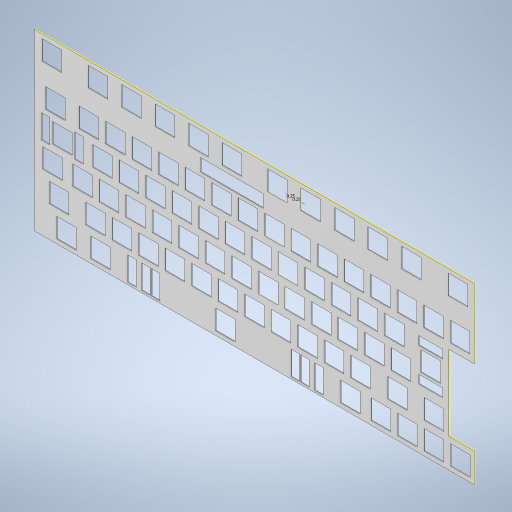
# Autodesk Inventor part: Plate
Saved by Autodesk Inventor 2024 (Build 280153000, 153)
## iProperties
Created: 2024-06-26
Part Number: Plate
Material: PET Plastic
Document SubType Name: Modeling
Designer: adam
Density: 1.541 g/cm^3
Appearance: Smooth - White
Author: adam
Autodesk Inventor part; units mm, degrees
(part 1 of 2)
ref_plane "YZ Plane" through (0, 0, 0) normal (1, 0, 0) x (0, 1, 0)
ref_plane "XZ Plane" through (0, 0, 0) normal (0, 1, 0) x (-1, 0, 0)
ref_plane "XY Plane" through (0, 0, 0) normal (0, 0, 1) x (1, 0, 0)
sketch "Keyswitch cut positions" plane through (0, 0, 0) normal (0, 0, 1) x (1, 0, 0)
  line L0 (0, 0) -> (315, 0)
  line L1 (315, -125) -> (0, -125)
  line L2 (0, -125) -> (0, 0)
  line L3 (5.475, -2.975) -> (19.525, -2.975)
  line L4 (19.525, -2.975) -> (19.525, -17.025)
  line L5 (19.525, -17.025) -> (5.475, -17.025)
  line L6 (5.475, -17.025) -> (5.475, -2.975)
  line L7 (5.475, -2.975) -> (19.525, -17.025) construction
  line L8 (19.525, -2.975) -> (5.475, -17.025) construction
  line L9 (38.475, -2.975) -> (52.525, -2.975)
  line L10 (52.525, -2.975) -> (52.525, -17.025)
  line L11 (52.525, -17.025) -> (38.475, -17.025)
  line L12 (38.475, -17.025) -> (38.475, -2.975)
  line L13 (38.475, -2.975) -> (52.525, -17.025) construction
  line L14 (52.525, -2.975) -> (38.475, -17.025) construction
  line L15 (62.475, -2.975) -> (76.525, -2.975)
  line L16 (76.525, -2.975) -> (76.525, -17.025)
  line L17 (76.525, -17.025) -> (62.475, -17.025)
  line L18 (62.475, -17.025) -> (62.475, -2.975)
  line L19 (62.475, -2.975) -> (76.525, -17.025) construction
  line L20 (76.525, -2.975) -> (62.475, -17.025) construction
  line L21 (86.475, -2.975) -> (100.525, -2.975)
  line L22 (100.525, -2.975) -> (100.525, -17.025)
  line L23 (100.525, -17.025) -> (86.475, -17.025)
  line L24 (86.475, -17.025) -> (86.475, -2.975)
  line L25 (86.475, -2.975) -> (100.525, -17.025) construction
  line L26 (100.525, -2.975) -> (86.475, -17.025) construction
  line L27 (110.475, -2.975) -> (124.525, -2.975)
  line L28 (124.525, -2.975) -> (124.525, -17.025)
  line L29 (124.525, -17.025) -> (110.475, -17.025)
  line L30 (110.475, -17.025) -> (110.475, -2.975)
  line L31 (110.475, -2.975) -> (124.525, -17.025) construction
  line L32 (124.525, -2.975) -> (110.475, -17.025) construction
  line L33 (134.475, -2.975) -> (148.525, -2.975)
  line L34 (148.525, -2.975) -> (148.525, -17.025)
  line L35 (148.525, -17.025) -> (134.475, -17.025)
  line L36 (134.475, -17.025) -> (134.475, -2.975)
  line L37 (134.475, -2.975) -> (148.525, -17.025) construction
  line L38 (148.525, -2.975) -> (134.475, -17.025) construction
  line L39 (166.975, -2.975) -> (181.025, -2.975)
  line L40 (181.025, -2.975) -> (181.025, -17.025)
  line L41 (181.025, -17.025) -> (166.975, -17.025)
  line L42 (166.975, -17.025) -> (166.975, -2.975)
  line L43 (166.975, -2.975) -> (181.025, -17.025) construction
  line L44 (181.025, -2.975) -> (166.975, -17.025) construction
  line L45 (190.975, -2.975) -> (205.025, -2.975)
  line L46 (205.025, -2.975) -> (205.025, -17.025)
  line L47 (205.025, -17.025) -> (190.975, -17.025)
  line L48 (190.975, -17.025) -> (190.975, -2.975)
  line L49 (190.975, -2.975) -> (205.025, -17.025) construction
  line L50 (205.025, -2.975) -> (190.975, -17.025) construction
  line L51 (214.975, -2.975) -> (229.025, -2.975)
  line L52 (229.025, -2.975) -> (229.025, -17.025)
  line L53 (229.025, -17.025) -> (214.975, -17.025)
  line L54 (214.975, -17.025) -> (214.975, -2.975)
  line L55 (214.975, -2.975) -> (229.025, -17.025) construction
  line L56 (229.025, -2.975) -> (214.975, -17.025) construction
  line L57 (238.975, -2.975) -> (253.025, -2.975)
  line L58 (253.025, -2.975) -> (253.025, -17.025)
  line L59 (253.025, -17.025) -> (238.975, -17.025)
  line L60 (238.975, -17.025) -> (238.975, -2.975)
  line L61 (238.975, -2.975) -> (253.025, -17.025) construction
  line L62 (253.025, -2.975) -> (238.975, -17.025) construction
  line L63 (262.975, -2.975) -> (277.025, -2.975)
  line L64 (277.025, -2.975) -> (277.025, -17.025)
  line L65 (277.025, -17.025) -> (262.975, -17.025)
  line L66 (262.975, -17.025) -> (262.975, -2.975)
  line L67 (262.975, -2.975) -> (277.025, -17.025) construction
  line L68 (277.025, -2.975) -> (262.975, -17.025) construction
  line L69 (296.475, -2.975) -> (310.525, -2.975)
  line L70 (310.525, -2.975) -> (310.525, -17.025)
  line L71 (310.525, -17.025) -> (296.475, -17.025)
  line L72 (296.475, -17.025) -> (296.475, -2.975)
  line L73 (296.475, -2.975) -> (310.525, -17.025) construction
  line L74 (310.525, -2.975) -> (296.475, -17.025) construction
  line L75 (7.975, -31.475) -> (22.025, -31.475)
  line L76 (22.025, -31.475) -> (22.025, -45.525)
  line L77 (22.025, -45.525) -> (7.975, -45.525)
  line L78 (7.975, -45.525) -> (7.975, -31.475)
  line L79 (7.975, -31.475) -> (22.025, -45.525) construction
  line L80 (22.025, -31.475) -> (7.975, -45.525) construction
  line L81 (31.975, -31.475) -> (46.025, -31.475)
  line L82 (46.025, -31.475) -> (46.025, -45.525)
  line L83 (46.025, -45.525) -> (31.975, -45.525)
  line L84 (31.975, -45.525) -> (31.975, -31.475)
  line L85 (31.975, -31.475) -> (46.025, -45.525) construction
  line L86 (46.025, -31.475) -> (31.975, -45.525) construction
  line L87 (50.975, -31.475) -> (65.025, -31.475)
  line L88 (65.025, -31.475) -> (65.025, -45.525)
  line L89 (65.025, -45.525) -> (50.975, -45.525)
  line L90 (50.975, -45.525) -> (50.975, -31.475)
  line L91 (50.975, -31.475) -> (65.025, -45.525) construction
  line L92 (65.025, -31.475) -> (50.975, -45.525) construction
  line L93 (69.975, -31.475) -> (84.025, -31.475)
  line L94 (84.025, -31.475) -> (84.025, -45.525)
  line L95 (84.025, -45.525) -> (69.975, -45.525)
  line L96 (69.975, -45.525) -> (69.975, -31.475)
  line L97 (69.975, -31.475) -> (84.025, -45.525) construction
  line L98 (84.025, -31.475) -> (69.975, -45.525) construction
  line L99 (88.975, -31.475) -> (103.025, -31.475)
  line L100 (103.025, -31.475) -> (103.025, -45.525)
  line L101 (103.025, -45.525) -> (88.975, -45.525)
  line L102 (88.975, -45.525) -> (88.975, -31.475)
  line L103 (88.975, -31.475) -> (103.025, -45.525) construction
  line L104 (103.025, -31.475) -> (88.975, -45.525) construction
  line L105 (107.975, -31.475) -> (122.025, -31.475)
  line L106 (122.025, -31.475) -> (122.025, -45.525)
  line L107 (122.025, -45.525) -> (107.975, -45.525)
  line L108 (107.975, -45.525) -> (107.975, -31.475)
  line L109 (107.975, -31.475) -> (122.025, -45.525) construction
  line L110 (122.025, -31.475) -> (107.975, -45.525) construction
  line L111 (126.975, -31.475) -> (141.025, -31.475)
  line L112 (141.025, -31.475) -> (141.025, -45.525)
  line L113 (141.025, -45.525) -> (126.975, -45.525)
  line L114 (126.975, -45.525) -> (126.975, -31.475)
  line L115 (126.975, -31.475) -> (141.025, -45.525) construction
  line L116 (141.025, -31.475) -> (126.975, -45.525) construction
  line L117 (145.975, -31.475) -> (160.025, -31.475)
  line L118 (160.025, -31.475) -> (160.025, -45.525)
  line L119 (160.025, -45.525) -> (145.975, -45.525)
  line L120 (145.975, -45.525) -> (145.975, -31.475)
  line L121 (145.975, -31.475) -> (160.025, -45.525) construction
  line L122 (160.025, -31.475) -> (145.975, -45.525) construction
  line L123 (164.975, -31.475) -> (179.025, -31.475)
  line L124 (179.025, -31.475) -> (179.025, -45.525)
  line L125 (179.025, -45.525) -> (164.975, -45.525)
  line L126 (164.975, -45.525) -> (164.975, -31.475)
  line L127 (164.975, -31.475) -> (179.025, -45.525) construction
  line L128 (179.025, -31.475) -> (164.975, -45.525) construction
  line L129 (183.975, -31.475) -> (198.025, -31.475)
  line L130 (198.025, -31.475) -> (198.025, -45.525)
  line L131 (198.025, -45.525) -> (183.975, -45.525)
  line L132 (183.975, -45.525) -> (183.975, -31.475)
  line L133 (183.975, -31.475) -> (198.025, -45.525) construction
  line L134 (198.025, -31.475) -> (183.975, -45.525) construction
  line L135 (202.975, -31.475) -> (217.025, -31.475)
  line L136 (217.025, -31.475) -> (217.025, -45.525)
  line L137 (217.025, -45.525) -> (202.975, -45.525)
  line L138 (202.975, -45.525) -> (202.975, -31.475)
  line L139 (202.975, -31.475) -> (217.025, -45.525) construction
  line L140 (217.025, -31.475) -> (202.975, -45.525) construction
  line L141 (221.975, -31.475) -> (236.025, -31.475)
  line L142 (236.025, -31.475) -> (236.025, -45.525)
  line L143 (236.025, -45.525) -> (221.975, -45.525)
  line L144 (221.975, -45.525) -> (221.975, -31.475)
  line L145 (221.975, -31.475) -> (236.025, -45.525) construction
  line L146 (236.025, -31.475) -> (221.975, -45.525) construction
  line L147 (240.975, -31.475) -> (255.025, -31.475)
  line L148 (255.025, -31.475) -> (255.025, -45.525)
  line L149 (255.025, -45.525) -> (240.975, -45.525)
  line L150 (240.975, -45.525) -> (240.975, -31.475)
  line L151 (240.975, -31.475) -> (255.025, -45.525) construction
  line L152 (255.025, -31.475) -> (240.975, -45.525) construction
  line L153 (259.975, -31.475) -> (274.025, -31.475)
  line L154 (274.025, -31.475) -> (274.025, -45.525)
  line L155 (274.025, -45.525) -> (259.975, -45.525)
  line L156 (259.975, -45.525) -> (259.975, -31.475)
  line L157 (259.975, -31.475) -> (274.025, -45.525) construction
  line L158 (274.025, -31.475) -> (259.975, -45.525) construction
  line L159 (278.975, -31.475) -> (293.025, -31.475)
  line L160 (293.025, -31.475) -> (293.025, -45.525)
  line L161 (293.025, -45.525) -> (278.975, -45.525)
  line L162 (278.975, -45.525) -> (278.975, -31.475)
  line L163 (278.975, -31.475) -> (293.025, -45.525) construction
  line L164 (293.025, -31.475) -> (278.975, -45.525) construction
  line L165 (297.975, -31.475) -> (312.025, -31.475)
  line L166 (312.025, -31.475) -> (312.025, -45.525)
  line L167 (312.025, -45.525) -> (297.975, -45.525)
  line L168 (297.975, -45.525) -> (297.975, -31.475)
  line L169 (297.975, -31.475) -> (312.025, -45.525) construction
  line L170 (312.025, -31.475) -> (297.975, -45.525) construction
  line L171 (12.975, -50.575) -> (27.025, -50.575)
  line L172 (27.025, -50.575) -> (27.025, -64.625)
  line L173 (27.025, -64.625) -> (12.975, -64.625)
  line L174 (12.975, -64.625) -> (12.975, -50.575)
  line L175 (12.975, -50.575) -> (27.025, -64.625) construction
  line L176 (27.025, -50.575) -> (12.975, -64.625) construction
  line L177 (41.725, -50.575) -> (55.775, -50.575)
  line L178 (55.775, -50.575) -> (55.775, -64.625)
  line L179 (55.775, -64.625) -> (41.725, -64.625)
  line L180 (41.725, -64.625) -> (41.725, -50.575)
  line L181 (41.725, -50.575) -> (55.775, -64.625) construction
  line L182 (55.775, -50.575) -> (41.725, -64.625) construction
  line L183 (60.725, -50.575) -> (74.775, -50.575)
  line L184 (74.775, -50.575) -> (74.775, -64.625)
  line L185 (74.775, -64.625) -> (60.725, -64.625)
  line L186 (60.725, -64.625) -> (60.725, -50.575)
  line L187 (60.725, -50.575) -> (74.775, -64.625) construction
  line L188 (74.775, -50.575) -> (60.725, -64.625) construction
  line L189 (79.725, -50.575) -> (93.775, -50.575)
  line L190 (93.775, -50.575) -> (93.775, -64.625)
  line L191 (93.775, -64.625) -> (79.725, -64.625)
  line L192 (79.725, -64.625) -> (79.725, -50.575)
  line L193 (79.725, -50.575) -> (93.775, -64.625) construction
  line L194 (93.775, -50.575) -> (79.725, -64.625) construction
  line L195 (98.725, -50.575) -> (112.775, -50.575)
  line L196 (112.775, -50.575) -> (112.775, -64.625)
  line L197 (112.775, -64.625) -> (98.725, -64.625)
  line L198 (98.725, -64.625) -> (98.725, -50.575)
  line L199 (98.725, -50.575) -> (112.775, -64.625) construction
  line L200 (112.775, -50.575) -> (98.725, -64.625) construction
  line L201 (117.725, -50.575) -> (131.775, -50.575)
  line L202 (131.775, -50.575) -> (131.775, -64.625)
  line L203 (131.775, -64.625) -> (117.725, -64.625)
  line L204 (117.725, -64.625) -> (117.725, -50.575)
  line L205 (117.725, -50.575) -> (131.775, -64.625) construction
  line L206 (131.775, -50.575) -> (117.725, -64.625) construction
  line L207 (136.725, -50.575) -> (150.775, -50.575)
  line L208 (150.775, -50.575) -> (150.775, -64.625)
  line L209 (150.775, -64.625) -> (136.725, -64.625)
  line L210 (136.725, -64.625) -> (136.725, -50.575)
  line L211 (136.725, -50.575) -> (150.775, -64.625) construction
  line L212 (150.775, -50.575) -> (136.725, -64.625) construction
  line L213 (155.725, -50.575) -> (169.775, -50.575)
  line L214 (169.775, -50.575) -> (169.775, -64.625)
  line L215 (169.775, -64.625) -> (155.725, -64.625)
  line L216 (155.725, -64.625) -> (155.725, -50.575)
  line L217 (155.725, -50.575) -> (169.775, -64.625) construction
  line L218 (169.775, -50.575) -> (155.725, -64.625) construction
  line L219 (174.725, -50.575) -> (188.775, -50.575)
  line L220 (188.775, -50.575) -> (188.775, -64.625)
  line L221 (188.775, -64.625) -> (174.725, -64.625)
  line L222 (174.725, -64.625) -> (174.725, -50.575)
  line L223 (174.725, -50.575) -> (188.775, -64.625) construction
  line L224 (188.775, -50.575) -> (174.725, -64.625) construction
  line L225 (193.725, -50.575) -> (207.775, -50.575)
  line L226 (207.775, -50.575) -> (207.775, -64.625)
  line L227 (207.775, -64.625) -> (193.725, -64.625)
  line L228 (193.725, -64.625) -> (193.725, -50.575)
  line L229 (193.725, -50.575) -> (207.775, -64.625) construction
  line L230 (207.775, -50.575) -> (193.725, -64.625) construction
  line L231 (212.725, -50.575) -> (226.775, -50.575)
  line L232 (226.775, -50.575) -> (226.775, -64.625)
  line L233 (226.775, -64.625) -> (212.725, -64.625)
  line L234 (212.725, -64.625) -> (212.725, -50.575)
  line L235 (212.725, -50.575) -> (226.775, -64.625) construction
  line L236 (226.775, -50.575) -> (212.725, -64.625) construction
  line L237 (231.725, -50.575) -> (245.775, -50.575)
  line L238 (245.775, -50.575) -> (245.775, -64.625)
  line L239 (245.775, -64.625) -> (231.725, -64.625)
  line L240 (231.725, -64.625) -> (231.725, -50.575)
  line L241 (231.725, -50.575) -> (245.775, -64.625) construction
  line L242 (245.775, -50.575) -> (231.725, -64.625) construction
  line L243 (250.725, -50.575) -> (264.775, -50.575)
  line L244 (264.775, -50.575) -> (264.775, -64.625)
  line L245 (264.775, -64.625) -> (250.725, -64.625)
  line L246 (250.725, -64.625) -> (250.725, -50.575)
  line L247 (250.725, -50.575) -> (264.775, -64.625) construction
  line L248 (264.775, -50.575) -> (250.725, -64.625) construction
  line L249 (276.95, -60.25) -> (291, -60.25)
  line L250 (291, -60.25) -> (291, -74.3)
  line L251 (291, -74.3) -> (276.95, -74.3)
  line L252 (276.95, -74.3) -> (276.95, -60.25)
  line L253 (276.95, -60.25) -> (291, -74.3) construction
  line L254 (291, -60.25) -> (276.95, -74.3) construction
  line L255 (5.975, -69.675) -> (20.025, -69.675)
  line L256 (20.025, -69.675) -> (20.025, -83.725)
  line L257 (20.025, -83.725) -> (5.975, -83.725)
  line L258 (5.975, -83.725) -> (5.975, -69.675)
  line L259 (5.975, -69.675) -> (20.025, -83.725) construction
  line L260 (20.025, -69.675) -> (5.975, -83.725) construction
  line L261 (27.475, -69.675) -> (41.525, -69.675)
  line L262 (41.525, -69.675) -> (41.525, -83.725)
  line L263 (41.525, -83.725) -> (27.475, -83.725)
  line L264 (27.475, -83.725) -> (27.475, -69.675)
  line L265 (27.475, -69.675) -> (41.525, -83.725) construction
  line L266 (41.525, -69.675) -> (27.475, -83.725) construction
  line L267 (46.475, -69.675) -> (60.525, -69.675)
  line L268 (60.525, -69.675) -> (60.525, -83.725)
  line L269 (60.525, -83.725) -> (46.475, -83.725)
  line L270 (46.475, -83.725) -> (46.475, -69.675)
  line L271 (46.475, -69.675) -> (60.525, -83.725) construction
  line L272 (60.525, -69.675) -> (46.475, -83.725) construction
  line L273 (65.475, -69.675) -> (79.525, -69.675)
  line L274 (79.525, -69.675) -> (79.525, -83.725)
  line L275 (79.525, -83.725) -> (65.475, -83.725)
  line L276 (65.475, -83.725) -> (65.475, -69.675)
  line L277 (65.475, -69.675) -> (79.525, -83.725) construction
  line L278 (79.525, -69.675) -> (65.475, -83.725) construction
  line L279 (84.475, -69.675) -> (98.525, -69.675)
  line L280 (98.525, -69.675) -> (98.525, -83.725)
  line L281 (98.525, -83.725) -> (84.475, -83.725)
  line L282 (84.475, -83.725) -> (84.475, -69.675)
  line L283 (84.475, -69.675) -> (98.525, -83.725) construction
  line L284 (98.525, -69.675) -> (84.475, -83.725) construction
  line L285 (103.475, -69.675) -> (117.525, -69.675)
  line L286 (117.525, -69.675) -> (117.525, -83.725)
  line L287 (117.525, -83.725) -> (103.475, -83.725)
  line L288 (103.475, -83.725) -> (103.475, -69.675)
  line L289 (103.475, -69.675) -> (117.525, -83.725) construction
  line L290 (117.525, -69.675) -> (103.475, -83.725) construction
  line L291 (122.475, -69.675) -> (136.525, -69.675)
  line L292 (136.525, -69.675) -> (136.525, -83.725)
  line L293 (136.525, -83.725) -> (122.475, -83.725)
  line L294 (122.475, -83.725) -> (122.475, -69.675)
  line L295 (122.475, -69.675) -> (136.525, -83.725) construction
  line L296 (136.525, -69.675) -> (122.475, -83.725) construction
  line L297 (141.475, -69.675) -> (155.525, -69.675)
  line L298 (155.525, -69.675) -> (155.525, -83.725)
  line L299 (155.525, -83.725) -> (141.475, -83.725)
  line L300 (141.475, -83.725) -> (141.475, -69.675)
  line L301 (141.475, -69.675) -> (155.525, -83.725) construction
  line L302 (155.525, -69.675) -> (141.475, -83.725) construction
  line L303 (160.475, -69.675) -> (174.525, -69.675)
  line L304 (174.525, -69.675) -> (174.525, -83.725)
  line L305 (174.525, -83.725) -> (160.475, -83.725)
  line L306 (160.475, -83.725) -> (160.475, -69.675)
  line L307 (160.475, -69.675) -> (174.525, -83.725) construction
  line L308 (174.525, -69.675) -> (160.475, -83.725) construction
  line L309 (179.475, -69.675) -> (193.525, -69.675)
  line L310 (193.525, -69.675) -> (193.525, -83.725)
  line L311 (193.525, -83.725) -> (179.475, -83.725)
  line L312 (179.475, -83.725) -> (179.475, -69.675)
  line L313 (179.475, -69.675) -> (193.525, -83.725) construction
  line L314 (193.525, -69.675) -> (179.475, -83.725) construction
  line L315 (198.475, -69.675) -> (212.525, -69.675)
  line L316 (212.525, -69.675) -> (212.525, -83.725)
  line L317 (212.525, -83.725) -> (198.475, -83.725)
  line L318 (198.475, -83.725) -> (198.475, -69.675)
  line L319 (198.475, -69.675) -> (212.525, -83.725) construction
  line L320 (212.525, -69.675) -> (198.475, -83.725) construction
  line L321 (217.475, -69.675) -> (231.525, -69.675)
  line L322 (231.525, -69.675) -> (231.525, -83.725)
  line L323 (231.525, -83.725) -> (217.475, -83.725)
  line L324 (217.475, -83.725) -> (217.475, -69.675)
  line L325 (217.475, -69.675) -> (231.525, -83.725) construction
  line L326 (231.525, -69.675) -> (217.475, -83.725) construction
  line L327 (236.475, -69.675) -> (250.525, -69.675)
  line L328 (250.525, -69.675) -> (250.525, -83.725)
  line L329 (250.525, -83.725) -> (236.475, -83.725)
  line L330 (236.475, -83.725) -> (236.475, -69.675)
  line L331 (236.475, -69.675) -> (250.525, -83.725) construction
  line L332 (250.525, -69.675) -> (236.475, -83.725) construction
  line L333 (255.475, -69.675) -> (269.525, -69.675)
  line L334 (269.525, -69.675) -> (269.525, -83.725)
  line L335 (269.525, -83.725) -> (255.475, -83.725)
  line L336 (255.475, -83.725) -> (255.475, -69.675)
  line L337 (255.475, -69.675) -> (269.525, -83.725) construction
  line L338 (269.525, -69.675) -> (255.475, -83.725) construction
  line L339 (10.725, -88.775) -> (24.775, -88.775)
  line L340 (24.775, -88.775) -> (24.775, -102.825)
  line L341 (24.775, -102.825) -> (10.725, -102.825)
  line L342 (10.725, -102.825) -> (10.725, -88.775)
  line L343 (10.725, -88.775) -> (24.775, -102.825) construction
  line L344 (24.775, -88.775) -> (10.725, -102.825) construction
  line L345 (36.725, -88.775) -> (50.775, -88.775)
  line L346 (50.775, -88.775) -> (50.775, -102.825)
  line L347 (50.775, -102.825) -> (36.725, -102.825)
  line L348 (36.725, -102.825) -> (36.725, -88.775)
  line L349 (36.725, -88.775) -> (50.775, -102.825) construction
  line L350 (50.775, -88.775) -> (36.725, -102.825) construction
  line L351 (55.725, -88.775) -> (69.775, -88.775)
  line L352 (69.775, -88.775) -> (69.775, -102.825)
  line L353 (69.775, -102.825) -> (55.725, -102.825)
  line L354 (55.725, -102.825) -> (55.725, -88.775)
  line L355 (55.725, -88.775) -> (69.775, -102.825) construction
  line L356 (69.775, -88.775) -> (55.725, -102.825) construction
  line L357 (74.725, -88.775) -> (88.775, -88.775)
  line L358 (88.775, -88.775) -> (88.775, -102.825)
  line L359 (88.775, -102.825) -> (74.725, -102.825)
  line L360 (74.725, -102.825) -> (74.725, -88.775)
  line L361 (74.725, -88.775) -> (88.775, -102.825) construction
  line L362 (88.775, -88.775) -> (74.725, -102.825) construction
  line L363 (93.725, -88.775) -> (107.775, -88.775)
  line L364 (107.775, -88.775) -> (107.775, -102.825)
  line L365 (107.775, -102.825) -> (93.725, -102.825)
  line L366 (93.725, -102.825) -> (93.725, -88.775)
  line L367 (93.725, -88.775) -> (107.775, -102.825) construction
  line L368 (107.775, -88.775) -> (93.725, -102.825) construction
  line L369 (112.725, -88.775) -> (126.775, -88.775)
  line L370 (126.775, -88.775) -> (126.775, -102.825)
  line L371 (126.775, -102.825) -> (112.725, -102.825)
  line L372 (112.725, -102.825) -> (112.725, -88.775)
  line L373 (112.725, -88.775) -> (126.775, -102.825) construction
  line L374 (126.775, -88.775) -> (112.725, -102.825) construction
  line L375 (131.725, -88.775) -> (145.775, -88.775)
  line L376 (145.775, -88.775) -> (145.775, -102.825)
  line L377 (145.775, -102.825) -> (131.725, -102.825)
  line L378 (131.725, -102.825) -> (131.725, -88.775)
  line L379 (131.725, -88.775) -> (145.775, -102.825) construction
  line L380 (145.775, -88.775) -> (131.725, -102.825) construction
  line L381 (150.725, -88.775) -> (164.775, -88.775)
  line L382 (164.775, -88.775) -> (164.775, -102.825)
  line L383 (164.775, -102.825) -> (150.725, -102.825)
  line L384 (150.725, -102.825) -> (150.725, -88.775)
  line L385 (150.725, -88.775) -> (164.775, -102.825) construction
  line L386 (164.775, -88.775) -> (150.725, -102.825) construction
  line L387 (169.725, -88.775) -> (183.775, -88.775)
  line L388 (183.775, -88.775) -> (183.775, -102.825)
  line L389 (183.775, -102.825) -> (169.725, -102.825)
  line L390 (169.725, -102.825) -> (169.725, -88.775)
  line L391 (169.725, -88.775) -> (183.775, -102.825) construction
  line L392 (183.775, -88.775) -> (169.725, -102.825) construction
  line L393 (188.725, -88.775) -> (202.775, -88.775)
  line L394 (202.775, -88.775) -> (202.775, -102.825)
  line L395 (202.775, -102.825) -> (188.725, -102.825)
  line L396 (188.725, -102.825) -> (188.725, -88.775)
  line L397 (188.725, -88.775) -> (202.775, -102.825) construction
  line L398 (202.775, -88.775) -> (188.725, -102.825) construction
  line L399 (207.725, -88.775) -> (221.775, -88.775)
  line L400 (221.775, -88.775) -> (221.775, -102.825)
  line L401 (221.775, -102.825) -> (207.725, -102.825)
  line L402 (207.725, -102.825) -> (207.725, -88.775)
  line L403 (207.725, -88.775) -> (221.775, -102.825) construction
  line L404 (221.775, -88.775) -> (207.725, -102.825) construction
  line L405 (226.725, -88.775) -> (240.775, -88.775)
  line L406 (240.775, -88.775) -> (240.775, -102.825)
  line L407 (240.775, -102.825) -> (226.725, -102.825)
  line L408 (226.725, -102.825) -> (226.725, -88.775)
  line L409 (226.725, -88.775) -> (240.775, -102.825) construction
  line L410 (240.775, -88.775) -> (226.725, -102.825) construction
  line L411 (252.975, -88.775) -> (267.025, -88.775)
  line L412 (267.025, -88.775) -> (267.025, -102.825)
  line L413 (267.025, -102.825) -> (252.975, -102.825)
  line L414 (252.975, -102.825) -> (252.975, -88.775)
  line L415 (252.975, -88.775) -> (267.025, -102.825) construction
  line L416 (267.025, -88.775) -> (252.975, -102.825) construction
  line L417 (279.225, -88.775) -> (293.275, -88.775)
  line L418 (293.275, -88.775) -> (293.275, -102.825)
  line L419 (293.275, -102.825) -> (279.225, -102.825)
  line L420 (279.225, -102.825) -> (279.225, -88.775)
  line L421 (279.225, -88.775) -> (293.275, -102.825) construction
  line L422 (293.275, -88.775) -> (279.225, -102.825) construction
  line L423 (15.975, -107.95) -> (30.025, -107.95)
  line L424 (30.025, -107.95) -> (30.025, -122)
  line L425 (30.025, -122) -> (15.975, -122)
  line L426 (15.975, -122) -> (15.975, -107.95)
  line L427 (15.975, -107.95) -> (30.025, -122) construction
  line L428 (30.025, -107.95) -> (15.975, -122) construction
  line L429 (40.475, -107.95) -> (54.525, -107.95)
  line L430 (54.525, -107.95) -> (54.525, -122)
  line L431 (54.525, -122) -> (40.475, -122)
  line L432 (40.475, -122) -> (40.475, -107.95)
  line L433 (40.475, -107.95) -> (54.525, -122) construction
  line L434 (54.525, -107.95) -> (40.475, -122) construction
  line L435 (129.825, -107.95) -> (143.875, -107.95)
  line L436 (143.875, -107.95) -> (143.875, -122)
  line L437 (143.875, -122) -> (129.825, -122)
  line L438 (129.825, -122) -> (129.825, -107.95)
  line L439 (129.825, -107.95) -> (143.875, -122) construction
  line L440 (143.875, -107.95) -> (129.825, -122) construction
  line L441 (219.225, -107.95) -> (233.275, -107.95)
  line L442 (233.275, -107.95) -> (233.275, -122)
  line L443 (233.275, -122) -> (219.225, -122)
  line L444 (219.225, -122) -> (219.225, -107.95)
  line L445 (219.225, -107.95) -> (233.275, -122) construction
  line L446 (233.275, -107.95) -> (219.225, -122) construction
  line L447 (241.225, -107.95) -> (255.275, -107.95)
  line L448 (255.275, -107.95) -> (255.275, -122)
  line L449 (255.275, -122) -> (241.225, -122)
  line L450 (241.225, -122) -> (241.225, -107.95)
  line L451 (241.225, -107.95) -> (255.275, -122) construction
  line L452 (255.275, -107.95) -> (241.225, -122) construction
  line L453 (260.225, -107.95) -> (274.275, -107.95)
  line L454 (274.275, -107.95) -> (274.275, -122)
  line L455 (274.275, -122) -> (260.225, -122)
  line L456 (260.225, -122) -> (260.225, -107.95)
  line L457 (260.225, -107.95) -> (274.275, -122) construction
  line L458 (274.275, -107.95) -> (260.225, -122) construction
  line L459 (279.225, -107.95) -> (293.275, -107.95)
  line L460 (293.275, -107.95) -> (293.275, -122)
  line L461 (293.275, -122) -> (279.225, -122)
  line L462 (279.225, -122) -> (279.225, -107.95)
  line L463 (279.225, -107.95) -> (293.275, -122) construction
  line L464 (293.275, -107.95) -> (279.225, -122) construction
  line L465 (298.225, -107.95) -> (312.275, -107.95)
  line L466 (312.275, -107.95) -> (312.275, -122)
  line L467 (312.275, -122) -> (298.225, -122)
  line L468 (298.225, -122) -> (298.225, -107.95)
  line L469 (298.225, -107.95) -> (312.275, -122) construction
  line L470 (312.275, -107.95) -> (298.225, -122) construction
  line L471 (136.85, -114.975) -> (203.85, -114.975) construction
  line L472 (315, -50) -> (297, -50)
  line L473 (297, -50) -> (297, -104)
  line L474 (297, -104) -> (315, -104)
  line L475 (315, 0) -> (315, -50)
  line L476 (315, -104) -> (315, -125)
  line L477 (119, -20) -> (164, -20)
  line L478 (164, -20) -> (164, -29)
  line L479 (164, -29) -> (119, -29)
  line L480 (119, -29) -> (119, -20)
  point P0 (12.5, -10)
  point P1 (45.5, -10)
  point P2 (69.5, -10)
  point P3 (93.5, -10)
  point P4 (117.5, -10)
  point P5 (141.5, -10)
  point P6 (174, -10)
  point P7 (198, -10)
  point P8 (222, -10)
  point P9 (246, -10)
  point P10 (270, -10)
  point P11 (303.5, -10)
  point P12 (15, -38.5)
  point P13 (39, -38.5)
  point P14 (58, -38.5)
  point P15 (77, -38.5)
  point P16 (96, -38.5)
  point P17 (115, -38.5)
  point P18 (134, -38.5)
  point P19 (153, -38.5)
  point P20 (172, -38.5)
  point P21 (191, -38.5)
  point P22 (210, -38.5)
  point P23 (229, -38.5)
  point P24 (248, -38.5)
  point P25 (267, -38.5)
  point P26 (286, -38.5)
  point P27 (305, -38.5)
  point P28 (20, -57.6)
  point P29 (48.75, -57.6)
  point P30 (67.75, -57.6)
  point P31 (86.75, -57.6)
  point P32 (105.75, -57.6)
  point P33 (124.75, -57.6)
  point P34 (143.75, -57.6)
  point P35 (162.75, -57.6)
  point P36 (181.75, -57.6)
  point P37 (200.75, -57.6)
  point P38 (219.75, -57.6)
  point P39 (238.75, -57.6)
  point P40 (257.75, -57.6)
  point P41 (283.975, -67.275)
  point P42 (296.597, -79.7566)
  point P43 (13, -76.7)
  point P44 (34.5, -76.7)
  point P45 (53.5, -76.7)
  point P46 (72.5, -76.7)
  point P47 (91.5, -76.7)
  point P48 (110.5, -76.7)
  point P49 (129.5, -76.7)
  point P50 (148.5, -76.7)
  point P51 (167.5, -76.7)
  point P52 (186.5, -76.7)
  point P53 (205.5, -76.7)
  point P54 (224.5, -76.7)
  point P55 (243.5, -76.7)
  point P56 (262.5, -76.7)
  point P57 (17.75, -95.8)
  point P58 (43.75, -95.8)
  point P59 (62.75, -95.8)
  point P60 (81.75, -95.8)
  point P61 (100.75, -95.8)
  point P62 (119.75, -95.8)
  point P63 (138.75, -95.8)
  point P64 (157.75, -95.8)
  point P65 (176.75, -95.8)
  point P66 (195.75, -95.8)
  point P67 (214.75, -95.8)
  point P68 (233.75, -95.8)
  point P69 (260, -95.8)
  point P70 (286.25, -95.8)
  point P71 (23, -114.975)
  point P72 (47.5, -114.975)
  point P73 (226.25, -114.975)
  point P74 (248.25, -114.975)
  point P75 (267.25, -114.975)
  point P76 (286.25, -114.975)
  point P77 (305.25, -114.975)
  point P78 (315, -62.5)
  dimension "d0" = 125
  dimension "d1" = 315
  dimension "d2" = 14.05
  dimension "d3" = 14.05
  dimension "d4" = 14.05
  dimension "d5" = 14.05
  dimension "d7" = 14.05
  dimension "d8" = 14.05
  dimension "d10" = 14.05
  dimension "d11" = 14.05
  dimension "d13" = 14.05
  dimension "d14" = 14.05
  dimension "d16" = 14.05
  dimension "d17" = 14.05
  dimension "d19" = 14.05
  dimension "d20" = 14.05
  dimension "d22" = 14.05
  dimension "d23" = 14.05
  dimension "d25" = 14.05
  dimension "d26" = 14.05
  dimension "d28" = 14.05
  dimension "d29" = 14.05
  dimension "d31" = 14.05
  dimension "d32" = 14.05
  dimension "d34" = 14.05
  dimension "d35" = 14.05
  dimension "d40" = 10
  dimension "d41" = 12.5
  dimension "d42" = 45.5
  dimension "d43" = 69.5
  dimension "d44" = 303.5
  dimension "d45" = 270
  dimension "d46" = 246
  dimension "d47" = 222
  dimension "d48" = 198
  dimension "d49" = 174
  dimension "d50" = 141.5
  dimension "d51" = 117.5
  dimension "d52" = 93.5
  dimension "d53" = 14.05
  dimension "d54" = 14.05
  dimension "d55" = 14.05
  dimension "d56" = 14.05
  dimension "d58" = 14.05
  dimension "d59" = 14.05
  dimension "d61" = 14.05
  dimension "d62" = 14.05
  dimension "d64" = 14.05
  dimension "d65" = 14.05
  dimension "d67" = 14.05
  dimension "d68" = 14.05
  dimension "d70" = 14.05
  dimension "d71" = 14.05
  dimension "d73" = 14.05
  dimension "d74" = 14.05
  dimension "d76" = 14.05
  dimension "d77" = 14.05
  dimension "d79" = 14.05
  dimension "d80" = 14.05
  dimension "d82" = 14.05
  dimension "d83" = 14.05
  dimension "d85" = 14.05
  dimension "d86" = 14.05
  dimension "d88" = 14.05
  constraints: 962 end point, 161 parallel, 156 midpoint, 86 perpendicular, 80 horizontal, 71 horizontal alignment, 1 collinear
  measures "d0" distance of L1.end L0.start
  measures "d1" distance of L0.start L0.end
  measures "d2" distance of L3.start L3.end
  measures "d3" distance of L5.end L3.start
  measures "d4" distance of L9.start L9.end
  measures "d5" distance of L11.end L9.start
  measures "d7" distance of L15.start L15.end
  measures "d8" distance of L17.end L15.start
  measures "d10" distance of L21.start L21.end
  measures "d11" distance of L23.end L21.start
  measures "d13" distance of L27.start L27.end
  measures "d14" distance of L29.end L27.start
  measures "d16" distance of L33.start L33.end
  measures "d17" distance of L35.end L33.start
  measures "d19" distance of L39.start L39.end
  measures "d20" distance of L41.end L39.start
  measures "d22" distance of L45.start L45.end
  measures "d23" distance of L47.end L45.start
  measures "d25" distance of L51.start L51.end
  measures "d26" distance of L53.end L51.start
  measures "d28" distance of L57.start L57.end
  measures "d29" distance of L59.end L57.start
  measures "d31" distance of L63.start L63.end
  measures "d32" distance of L65.end L63.start
  measures "d34" distance of L69.start L69.end
  measures "d35" distance of L71.end L69.start
  measures "d40" distance from line of point (12.5, -10) L0
  measures "d41" distance from line of L2 point (12.5, -10)
  measures "d42" distance from line of L2 point (45.5, -10)
  measures "d43" distance from line of L2 point (69.5, -10)
  measures "d44" distance from line of L2 point (303.5, -10)
  measures "d45" distance from line of L2 point (270, -10)
  measures "d46" distance from line of L2 point (246, -10)
  measures "d47" distance from line of L2 point (222, -10)
  measures "d48" distance from line of L2 point (198, -10)
  measures "d49" distance from line of L2 point (174, -10)
  measures "d50" distance from line of L2 point (141.5, -10)
  measures "d51" distance from line of L2 point (117.5, -10)
  measures "d52" distance from line of L2 point (93.5, -10)
  measures "d53" distance of L75.start L75.end
  measures "d54" distance of L77.end L75.start
  measures "d55" distance of L84.end L81.end
  measures "d56" distance of L83.end L84.end
  measures "d58" distance of L90.end L87.end
  measures "d59" distance of L89.end L90.end
  measures "d61" distance of L96.end L93.end
  measures "d62" distance of L95.end L96.end
  measures "d64" distance of L102.end L99.end
  measures "d65" distance of L101.end L102.end
  measures "d67" distance of L108.end L105.end
  measures "d68" distance of L107.end L108.end
  measures "d70" distance of L114.end L111.end
  measures "d71" distance of L113.end L114.end
  measures "d73" distance of L120.end L117.end
  measures "d74" distance of L119.end L120.end
  measures "d76" distance of L126.end L123.end
  measures "d77" distance of L125.end L126.end
  measures "d79" distance of L132.end L129.end
  measures "d80" distance of L131.end L132.end
  measures "d82" distance of L138.end L135.end
  measures "d83" distance of L137.end L138.end
  measures "d85" distance of L144.end L141.end
  measures "d86" distance of L143.end L144.end
  measures "d88" distance of L150.end L147.end
extrude "Keyswitches" add sketch "Keyswitch cut positions" against normal blind 0.5
sketch "Stabilizer cut positions" plane through (0, 0, 0) normal (0, 0, 1) x (1, 0, 0)
  line L0 (12.975, -50.575) -> (27.025, -50.575) construction
  line L1 (27.025, -50.575) -> (27.025, -64.625) construction
  line L2 (27.025, -64.625) -> (12.975, -64.625) construction
  line L3 (12.975, -64.625) -> (12.975, -50.575) construction
  line L4 (276.95, -60.25) -> (291, -60.25) construction
  line L5 (291, -60.25) -> (291, -74.3) construction
  line L6 (291, -74.3) -> (276.95, -74.3) construction
  line L7 (276.95, -74.3) -> (276.95, -60.25) construction
  line L8 (129.825, -107.95) -> (143.875, -107.95) construction
  line L9 (143.875, -107.95) -> (143.875, -122) construction
  line L10 (129.825, -122) -> (129.825, -107.95) construction
  line L11 (143.875, -122) -> (129.825, -122) construction
  line L12 (4.975, -49.075) -> (11.025, -49.075)
  line L13 (11.025, -49.075) -> (11.025, -66.125)
  line L14 (11.025, -66.125) -> (4.975, -66.125)
  line L15 (4.975, -66.125) -> (4.975, -49.075)
  line L16 (8, -49.075) -> (8, -66.125) construction
  line L17 (20, -50.575) -> (20, -64.625) construction
  line L18 (12.975, -57.6) -> (27.025, -57.6) construction
  line L19 (136.85, -107.95) -> (136.85, -122) construction
  line L20 (143.875, -114.975) -> (129.825, -114.975) construction
  line L21 (283.975, -60.25) -> (283.975, -74.3) construction
  line L22 (291, -67.275) -> (276.95, -67.275) construction
  line L23 (4.975, -57.6) -> (11.025, -57.6) construction
  line L24 (28.975, -49.075) -> (35.025, -49.075)
  line L25 (35.025, -49.075) -> (35.025, -66.125)
  line L26 (35.025, -66.125) -> (28.975, -66.125)
  line L27 (28.975, -66.125) -> (28.975, -49.075)
  line L28 (32, -49.075) -> (32, -66.125) construction
  line L29 (28.975, -57.6) -> (35.025, -57.6) construction
  line L30 (66.825, -106.45) -> (72.875, -106.45)
  line L31 (72.875, -106.45) -> (72.875, -123.5)
  line L32 (72.875, -123.5) -> (66.825, -123.5)
  line L33 (66.825, -123.5) -> (66.825, -106.45)
  line L34 (69.85, -106.45) -> (69.85, -123.5) construction
  line L35 (66.825, -114.975) -> (72.875, -114.975) construction
  line L36 (76.825, -106.45) -> (82.875, -106.45)
  line L37 (82.875, -106.45) -> (82.875, -123.5)
  line L38 (82.875, -123.5) -> (76.825, -123.5)
  line L39 (76.825, -123.5) -> (76.825, -106.45)
  line L40 (79.85, -106.45) -> (79.85, -123.5) construction
  line L41 (76.825, -114.975) -> (82.875, -114.975) construction
  line L42 (83.825, -106.45) -> (89.875, -106.45)
  line L43 (89.875, -106.45) -> (89.875, -123.5)
  line L44 (89.875, -123.5) -> (83.825, -123.5)
  line L45 (83.825, -123.5) -> (83.825, -106.45)
  line L46 (86.85, -106.45) -> (86.85, -123.5) construction
  line L47 (83.825, -114.975) -> (89.875, -114.975) construction
  line L48 (200.825, -106.45) -> (206.875, -106.45)
  line L49 (206.875, -106.45) -> (206.875, -123.5)
  line L50 (206.875, -123.5) -> (200.825, -123.5)
  line L51 (200.825, -123.5) -> (200.825, -106.45)
  line L52 (203.85, -106.45) -> (203.85, -123.5) construction
  line L53 (200.825, -114.975) -> (206.875, -114.975) construction
  line L54 (190.825, -106.45) -> (196.875, -106.45)
  line L55 (196.875, -106.45) -> (196.875, -123.5)
  line L56 (196.875, -123.5) -> (190.825, -123.5)
  line L57 (190.825, -123.5) -> (190.825, -106.45)
  line L58 (193.85, -106.45) -> (193.85, -123.5) construction
  line L59 (190.825, -114.975) -> (196.875, -114.975) construction
  line L60 (183.825, -106.45) -> (189.875, -106.45)
  line L61 (189.875, -106.45) -> (189.875, -123.5)
  line L62 (189.875, -123.5) -> (183.825, -123.5)
  line L63 (183.825, -123.5) -> (183.825, -106.45)
  line L64 (186.85, -106.45) -> (186.85, -123.5) construction
  line L65 (183.825, -114.975) -> (189.875, -114.975) construction
  line L66 (275.45, -52.25) -> (292.5, -52.25)
  line L67 (292.5, -52.25) -> (292.5, -58.3)
  line L68 (292.5, -58.3) -> (275.45, -58.3)
  line L69 (275.45, -58.3) -> (275.45, -52.25)
  line L70 (283.975, -52.25) -> (283.975, -58.3) construction
  line L71 (275.45, -55.275) -> (292.5, -55.275) construction
  line L72 (275.45, -76.25) -> (292.5, -76.25)
  line L73 (292.5, -76.25) -> (292.5, -82.3)
  line L74 (292.5, -82.3) -> (275.45, -82.3)
  line L75 (275.45, -82.3) -> (275.45, -76.25)
  line L76 (283.975, -76.25) -> (283.975, -82.3) construction
  line L77 (275.45, -79.275) -> (292.5, -79.275) construction
  point P0 (0, 0)
  dimension "d472" = 17.05
  dimension "d473" = 6.05
  dimension "d474" = 17.05
  dimension "d475" = 6.05
  dimension "d478" = 17.05
  dimension "d479" = 6.05
  dimension "d482" = 17.05
  dimension "d483" = 6.05
  dimension "d486" = 17.05
  dimension "d487" = 6.05
  dimension "d490" = 17.05
  dimension "d491" = 6.05
  dimension "d494" = 17.05
  dimension "d495" = 6.05
  dimension "d498" = 17.05
  dimension "d499" = 6.05
  dimension "d502" = 6.05
  dimension "d503" = 17.05
  dimension "d504" = 6.05
  dimension "d505" = 17.05
  dimension "d508" = 12
  dimension "d509" = 12
  dimension "d510" = 50
  dimension "d511" = 50
  dimension "d512" = 57
  dimension "d513" = 57
  dimension "d514" = 67
  dimension "d515" = 67
  dimension "d516" = 12
  dimension "d517" = 12
  constraints: 132 end point, 52 midpoint, 20 parallel, 10 collinear, 10 horizontal, 10 perpendicular
  measures "d472" distance of L14.end L12.start
  measures "d473" distance of L12.start L12.end
  measures "d474" distance of L26.end L27.end
  measures "d475" distance of L27.end L25.start
  measures "d478" distance of L32.end L33.end
  measures "d479" distance of L33.end L31.start
  measures "d482" distance of L38.end L39.end
  measures "d483" distance of L39.end L37.start
  measures "d486" distance of L44.end L45.end
  measures "d487" distance of L45.end L43.start
  measures "d490" distance of L50.end L51.end
  measures "d491" distance of L51.end L49.start
  measures "d494" distance of L56.end L57.end
  measures "d495" distance of L57.end L55.start
  measures "d498" distance of L62.end L63.end
  measures "d499" distance of L63.end L61.start
  measures "d502" distance of L68.end L66.start
  measures "d503" distance of L66.start L66.end
  measures "d504" distance of L75.start L75.end
  measures "d505" distance of L75.end L72.end
  measures "d508" distance between parallel lines of L22 L71
  measures "d509" distance between parallel lines of L22 L77
  measures "d510" distance between parallel lines of L19 L46
  measures "d511" distance between parallel lines of L64 L19
  measures "d512" distance between parallel lines of L19 L40
  measures "d513" distance between parallel lines of L58 L19
  measures "d514" distance between parallel lines of L19 L34
  measures "d515" distance between parallel lines of L52 L19
  measures "d516" distance between parallel lines of L17 L16
  measures "d517" distance between parallel lines of L28 L17
extrude "Stabilizers" cut sketch "Stabilizer cut positions" against normal up to surface (0.5 mm away)
sketch "Locating pin positions" plane through (0, 0, 0) normal (0, 0, 1) x (1, 0, 0)
  circle A0 centre (105, -10) radius 1.5
  circle A1 centre (58, -57) radius 1.5
  circle A2 centre (191, -58) radius 1.5
  circle A3 centre (270, -58) radius 1.5
  circle A4 centre (238, -115) radius 1.5
  circle A5 centre (58, -115) radius 1.5
  circle A6 centre (210, -10) radius 1.5
  line L0 (315, 0) -> (0, 0) projected
  line L1 (0, 0) -> (0, -125) projected
  point P0 (157.5, 0)
  dimension "d520" = 3
  dimension "d527" = 10
  dimension "d528" = 105
  dimension "d529" = 10
  dimension "d530" = 210
  dimension "d531" = 58
  dimension "d532" = 57
  dimension "d533" = 58
  dimension "d534" = 191
  dimension "d535" = 58
  dimension "d536" = 270
  dimension "d537" = 115
  dimension "d538" = 58
  dimension "d539" = 238
  dimension "d540" = 115
  constraints: 7 centre point, 6 equal radius, 1 midpoint
  measures "d520" diameter of A0
  measures "d527" distance from line of L0 A0.centre
  measures "d528" distance from line of L1 A0.centre
  measures "d529" vertical distance of point (157.5, 0) A6.centre
  measures "d530" distance from line of L1 A6.centre
  measures "d531" distance from line of L1 A1.centre
  measures "d532" distance from line of A1.centre L0
  measures "d533" distance from line of L0 A2.centre
  measures "d534" distance from line of A2.centre L1
  measures "d535" distance from line of L0 A3.centre
  measures "d536" distance from line of L1 A3.centre
  measures "d537" distance from line of A5.centre L0
  measures "d538" distance from line of A5.centre L1
  measures "d539" distance from line of A4.centre L1
  measures "d540" distance from line of A4.centre L0
extrude "Locating pins" add sketch "Locating pin positions" against normal blind 2.5
chamfer "Chamfer1" distance 1 angle 45 7 edges at (208.5, -10, -2.5) (103.5, -10, -2.5) (268.5, -58, -2.5) (189.5, -58, -2.5) (56.5, -57, -2.5) (236.5, -115, -2.5) (56.5, -115, -2.5)
sketch "Sketch9" plane through (0, 0, -0.5) normal (0, 0, -1) x (-1, 0, 0)
  line L0 (0, 0) -> (-315, 0) projected
  line L1 (-315, 0) -> (-315, -50) projected
  line L2 (-315, -50) -> (-297, -50) projected
  line L3 (-297, -50) -> (-297, -104) projected
  line L4 (-297, -104) -> (-315, -104) projected
  line L5 (-315, -104) -> (-315, -125) projected
  line L6 (-315, -125) -> (0, -125) projected
  line L7 (0, -125) -> (0, 0) projected
  line L8 (-169.725, -88.775) -> (-169.725, -102.825) construction
  line L9 (-164.775, -102.825) -> (-164.775, -88.775) construction
  line L10 (-183.775, -88.775) -> (-169.725, -88.775) construction
  line L11 (-160.475, -83.725) -> (-174.525, -83.725) construction
  line L12 (-174.525, -83.725) -> (-174.525, -69.675) construction
  line L13 (-179.475, -69.675) -> (-179.475, -83.725) construction
  line L14 (-174.725, -64.625) -> (-188.775, -64.625) construction
  line L15 (-174.725, -50.575) -> (-174.725, -64.625) construction
  line L16 (-169.775, -64.625) -> (-169.775, -50.575) construction
  line L17 (-188.775, -50.575) -> (-174.725, -50.575) construction
  line L18 (-164.975, -45.525) -> (-179.025, -45.525) construction
  line L19 (-179.025, -45.525) -> (-179.025, -31.475) construction
  line L20 (-183.975, -31.475) -> (-183.975, -45.525) construction
  line L21 (-179.025, -31.475) -> (-164.975, -31.475) construction
  line L22 (-166.975, -17.025) -> (-181.025, -17.025) construction
  line L23 (-181.025, -17.025) -> (-181.025, -2.975) construction
  line L24 (-190.975, -2.975) -> (-190.975, -17.025) construction
  line L25 (-186, 0) -> (-186, -24.25) construction
  line L26 (-186, -24.25) -> (-181.5, -24.25) construction
  line L27 (-181.5, -24.25) -> (-181.5, -48.05) construction
  line L28 (-181.5, -48.05) -> (-172.25, -48.05) construction
  line L29 (-172.25, -48.05) -> (-172.25, -67.15) construction
  line L30 (-172.25, -67.15) -> (-177, -67.15) construction
  line L31 (-177, -67.15) -> (-177, -86.25) construction
  line L32 (-177, -86.25) -> (-167.25, -86.25) construction
  line L33 (-167.25, -86.25) -> (-167.25, -125) construction
  line L34 (-190.975, -17.025) -> (-186, -17.025) construction
  line L35 (-186, -17.025) -> (-181.025, -17.025) construction
  line L36 (-183.975, -31.475) -> (-181.5, -31.475) construction
  line L37 (-179.025, -31.475) -> (-181.5, -31.475) construction
  line L38 (-179.025, -45.525) -> (-179.025, -48.05) construction
  line L39 (-179.025, -48.05) -> (-179.025, -50.575) construction
  line L40 (-174.725, -50.575) -> (-172.25, -50.575) construction
  line L41 (-172.25, -50.575) -> (-169.775, -50.575) construction
  line L42 (-174.725, -64.625) -> (-174.725, -67.15) construction
  line L43 (-179.475, -69.675) -> (-193.525, -69.675) construction
  line L44 (-179.475, -69.675) -> (-177, -69.675) construction
  line L45 (-174.525, -69.675) -> (-177, -69.675) construction
  line L46 (-174.525, -83.725) -> (-174.525, -86.25) construction
  line L47 (-174.525, -86.25) -> (-174.525, -88.775) construction
  line L48 (-169.725, -88.775) -> (-167.25, -88.775) construction
  line L49 (-164.775, -88.775) -> (-167.25, -88.775) construction
  line L50 (-174.525, -69.675) -> (-160.475, -69.675) construction
  line L51 (-174.725, -67.15) -> (-174.725, -69.675) construction
  line L52 (-181.025, -17.025) -> (-181.025, -24.25) construction
  line L53 (-181.025, -24.25) -> (-181.025, -31.475) construction
  line L54 (-186.25, 0) -> (-186.25, -24.5)
  line L55 (-186.25, -24.5) -> (-181.75, -24.5)
  line L56 (-181.75, -24.5) -> (-181.75, -48.3)
  line L57 (-181.75, -48.3) -> (-172.5, -48.3)
  line L58 (-172.5, -48.3) -> (-172.5, -66.9)
  line L59 (-172.5, -66.9) -> (-177.25, -66.9)
  line L60 (-177.25, -66.9) -> (-177.25, -86.5)
  line L61 (-177.25, -86.5) -> (-167.5, -86.5)
  line L62 (-167.5, -86.5) -> (-167.5, -125)
  line L63 (-185.75, 0) -> (-185.75, -24)
  line L64 (-185.75, -24) -> (-181.25, -24)
  line L65 (-181.25, -24) -> (-181.25, -47.8)
  line L66 (-181.25, -47.8) -> (-172, -47.8)
  line L67 (-172, -47.8) -> (-172, -67.4)
  line L68 (-172, -67.4) -> (-176.75, -67.4)
  line L69 (-176.75, -67.4) -> (-176.75, -86)
  line L70 (-176.75, -86) -> (-167, -86)
  line L71 (-167, -86) -> (-167, -125)
  dimension "d548" = 0.25
  dimension "d549" = 0.25
  constraints: 90 end point, 27 perpendicular, 20 point on line, 14 collinear, 1 parallel, 1 vertical, 16 other
  measures "d548" distance between parallel lines of L25 L54
  measures "d549" distance between parallel lines of L25 L63
equation "\"d2\" = kd"
equation "\"d3\" = kd"
equation "\"d53\" = kd"
equation "\"d54\" = kd"
equation "\"kd\" = 14.05"
equation "\"d6\" = 14.05"
equation "\"d9\" = 14.05"
equation "\"d12\" = 14.05"
equation "\"d15\" = 14.05"
equation "\"d18\" = 14.05"
equation "\"d21\" = 14.05"
equation "\"d24\" = 14.05"
equation "\"d27\" = 14.05"
equation "\"d30\" = 14.05"
equation "\"d33\" = 14.05"
equation "\"d36\" = 14.05"
equation "\"d39\" = 14.05"
equation "\"d57\" = 14.05"
equation "\"d60\" = 14.05"
equation "\"d63\" = 14.05"
equation "\"d66\" = 14.05"
equation "\"d69\" = 14.05"
equation "\"d72\" = 14.05"
equation "\"d75\" = 14.05"
equation "\"d78\" = 14.05"
equation "\"d81\" = 14.05"
equation "\"d84\" = 14.05"
equation "\"d87\" = 14.05"
equation "\"d90\" = 14.05"
equation "\"d93\" = 14.05"
equation "\"d96\" = 14.05"
equation "\"d99\" = 14.05"
equation "\"d121\" = 14.05"
equation "\"d124\" = 14.05"
equation "\"d127\" = 14.05"
equation "\"d130\" = 14.05"
equation "\"d133\" = 14.05"
equation "\"d136\" = 14.05"
equation "\"d139\" = 14.05"
equation "\"d142\" = 14.05"
equation "\"d145\" = 14.05"
equation "\"d148\" = 14.05"
equation "\"d151\" = 14.05"
equation "\"d154\" = 14.05"
equation "\"stabh\" = 6.05"
equation "\"stabv\" = 17.05"
equation "\"d177\" = 6.05"
equation "\"d178\" = 17.05"
equation "\"d183\" = 6.05"
equation "\"d184\" = 17.05"
equation "\"d187\" = 6.05"
equation "\"d188\" = 17.05"
equation "\"d197\" = 14.05"
equation "\"d200\" = 14.05"
equation "\"d203\" = 14.05"
equation "\"d206\" = 14.05"
equation "\"d209\" = 14.05"
equation "\"d212\" = 14.05"
equation "\"d215\" = 14.05"
equation "\"d218\" = 14.05"
equation "\"d221\" = 14.05"
equation "\"d224\" = 14.05"
equation "\"d227\" = 14.05"
equation "\"d230\" = 14.05"
equation "\"d233\" = 14.05"
equation "\"d255\" = 14.05"
equation "\"d258\" = 14.05"
equation "\"d261\" = 14.05"
equation "\"d264\" = 14.05"
equation "\"d267\" = 14.05"
equation "\"d270\" = 14.05"
equation "\"d273\" = 14.05"
equation "\"d276\" = 14.05"
equation "\"d279\" = 14.05"
equation "\"d282\" = 14.05"
equation "\"d285\" = 14.05"
equation "\"d288\" = 14.05"
equation "\"d291\" = 14.05"
equation "\"d311\" = 14.05"
equation "\"d314\" = 14.05"
equation "\"d317\" = 14.05"